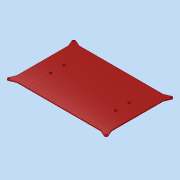
# Autodesk Inventor part: vna_mount
Saved by Autodesk Inventor 2022 (Build 260153000, 153)
## iProperties
Created: 2020-10-01
Part Number: vna_mount
Material: Generic
Document SubType Name: Modeling
Designer: nnico
Density: 1 g/cm^3
Appearance: Red
Author: nnico
Autodesk Inventor part; units mm, degrees
ref_plane "YZ Plane" through (0, 0, 0) normal (1, 0, 0) x (0, 1, 0)
ref_plane "XZ Plane" through (0, 0, 0) normal (0, 1, 0) x (-1, 0, 0)
ref_plane "XY Plane" through (0, 0, 0) normal (0, 0, 1) x (1, 0, 0)
sketch "Sketch1" plane through (0, 0, 0) normal (0, 1, 0) x (-1, 0, 0)
  line L0 (175, -115) -> (-175, -115)
  line L1 (-175, -115) -> (-175, 115)
  line L2 (-175, 115) -> (175, 115)
  line L3 (175, 115) -> (175, -115)
  line L4 (0, -115) -> (0, 115) construction
  line L5 (175, 0) -> (-175, 0) construction
  point P0 (0, 0)
  point P1 (0, 0)
  dimension "d0" = 350
  dimension "d1" = 230
  constraints: 12 end point, 5 midpoint, 2 parallel, 1 coincident, 1 horizontal, 1 perpendicular
  measures "d0" distance of L1.end L2.end
  measures "d1" distance of L0.end L1.end
extrude "Extrusion1" add sketch "Sketch1" along normal blind 3
sketch "Sketch2" plane through (0, 0, 0) normal (0, -1, 0) x (1, 0, 0)
  line L0 (175, -115) -> (-175, -115) construction
  line L1 (0, -115) -> (0, 115) construction
  line L2 (-175, 115) -> (175, 115) construction
  line L3 (130, -40) -> (110, -40)
  line L4 (110, -40) -> (110, 40)
  line L5 (110, 40) -> (130, 40)
  line L6 (130, 40) -> (130, -40)
  line L7 (130, 0) -> (110, 0) construction
  line L8 (0, 0) -> (175, 0) construction
  line L9 (175, 115) -> (175, -115) construction
  line L10 (-130, -40) -> (-110, -40)
  line L11 (-110, -40) -> (-110, 40)
  line L12 (-110, 40) -> (-130, 40)
  line L13 (-130, 40) -> (-130, -40)
  dimension "d4" = 20
  dimension "d5" = 80
  dimension "d6" = 220
  constraints: 22 end point, 5 midpoint, 4 symmetric about line, 2 parallel, 1 collinear, 1 horizontal, 1 perpendicular
  measures "d4" distance of L3.start L3.end
  measures "d5" distance of L5.end L3.start
  measures "d6" diameter of L3.end L1
extrude "Extrusion2" add sketch "Sketch2" along normal blind 10
sketch "Sketch3" plane through (0, -10, 0) normal (0, -1, 0) x (1, 0, 0)
  line L0 (175, 115) -> (-175, 115) construction
  line L1 (0, 115) -> (0, -115) construction
  line L2 (175, -115) -> (-175, -115) construction
  line L3 (0, 0) -> (-175, 0) construction
  line L4 (-175, 115) -> (-175, -115) construction
  line L5 (-110, 40) -> (-130, 40) construction
  line L6 (-120, 40) -> (-120, -40) construction
  line L7 (-130, -40) -> (-110, -40) construction
  circle A0 centre (-120, 25) radius 2.75
  circle A1 centre (-120, -25) radius 2.75
  circle A2 centre (120, 25) radius 2.75
  circle A3 centre (120, -25) radius 2.75
  dimension "d9" = 5.5
  dimension "d10" = 15
  constraints: 6 end point, 5 midpoint, 4 centre point, 3 symmetric about line, 1 point on line, 3 other
  measures "d9" diameter of A0
  measures "d10" distance from line of L5 A0.centre
extrude "Extrusion3" cut sketch "Sketch3" against normal up to next
sketch "Sketch4" plane through (0, 0, 0) normal (0, -1, 0) x (1, 0, 0)
  line L0 (110, 40) -> (110, -40) construction
  line L1 (110, 0) -> (-110, 0) construction
  line L2 (-110, -40) -> (-110, 40) construction
  line L3 (110, 15) -> (-110, 15)
  line L4 (-110, 15) -> (-110, 20)
  line L5 (-110, 20) -> (110, 20)
  line L6 (110, 20) -> (110, 15)
  line L7 (110, -15) -> (-110, -15)
  line L8 (-110, -15) -> (-110, -20)
  line L9 (-110, -20) -> (110, -20)
  line L10 (110, -20) -> (110, -15)
  point P0 (0, 0)
  dimension "d13" = 5
  dimension "d14" = 30
  constraints: 18 end point, 4 symmetric about line, 2 midpoint, 2 parallel, 2 point on line, 1 horizontal, 1 perpendicular
  measures "d13" distance of L3.end L4.end
  measures "d14" diameter of L3 L1
extrude "Extrusion4" add sketch "Sketch4" along normal blind 5
fillet "Fillet1" radius 10 6 edges at (120, 0, 40) (130, 0, 0) (120, 0, -40) (-120, 0, 40) (-130, 0, 0) (-120, 0, -40)
fillet "Fillet2" radius 5 4 edges at (0, 0, 20) (0, 0, -15) (0, 0, 15) (0, 0, -20)
sketch "Sketch5" plane through (0, 3, 0) normal (0, 1, 0) x (1, 0, 0)
  line L0 (-175, -115) -> (-175, 115) construction
  line L1 (-175, 0) -> (175, 0) construction
  line L2 (175, -115) -> (175, 115) construction
  line L3 (175, -115) -> (-175, -115) construction
  line L4 (0, -115) -> (0, 115) construction
  line L5 (-175, 115) -> (175, 115) construction
  circle A0 centre (-120, 25) radius 2.75 projected
  circle A1 centre (-120, 25) radius 4.5
  circle A2 centre (-120, -25) radius 4.5
  circle A3 centre (120, 25) radius 4.5
  circle A4 centre (120, -25) radius 4.5
  point P0 (0, 0)
  dimension "d19" = 9
  constraints: 4 centre point, 4 end point, 4 midpoint, 3 symmetric about line, 1 coincident, 3 other
  measures "d19" diameter of A1
extrude "Extrusion5" cut sketch "Sketch5" against normal blind 6
sketch "Sketch6" plane through (0, 3, 0) normal (0, 1, 0) x (1, 0, 0)
  line L0 (175, 115) -> (-175, 115) construction
  line L1 (0, 115) -> (0, -115) construction
  line L2 (175, -115) -> (-175, -115) construction
  line L3 (-175, 115) -> (-175, -115) construction
  line L4 (-175, 0) -> (175, 0) construction
  line L5 (175, -115) -> (175, 115) construction
  circle A0 centre (-179, 119) radius 6
  line L6 (-175, 115) -> (-179, 115) construction
  line L7 (-179, 115) -> (-179, 119) construction
  line L8 (-179, 119) -> (-175, 119) construction
  line L9 (-175, 119) -> (-175, 115) construction
  line L10 (-155, 115) -> (-175.4528, 123.8392)
  line L11 (-175, 95) -> (-183.0203, 114.5461)
  line L12 (-175, 95) -> (-175, 115)
  line L13 (-155, 115) -> (-175, 115)
  circle A1 centre (-179, -119) radius 6
  line L14 (-155, -115) -> (-175.4528, -123.8392)
  line L15 (-175, -95) -> (-183.0203, -114.5461)
  line L16 (-175, -95) -> (-175, -115)
  line L17 (-155, -115) -> (-175, -115)
  circle A2 centre (179, 119) radius 6
  line L18 (155, 115) -> (175.4528, 123.8392)
  line L19 (175, 95) -> (183.0203, 114.5461)
  line L20 (175, 95) -> (175, 115)
  line L21 (155, 115) -> (175, 115)
  line L22 (175, -95) -> (183.0203, -114.5461)
  circle A3 centre (179, -119) radius 6
  line L23 (155, -115) -> (175.4528, -123.8392)
  line L24 (155, -115) -> (175, -115)
  line L25 (175, -95) -> (175, -115)
  circle A4 centre (179, -119) radius 2.75
  circle A5 centre (179, 119) radius 2.75
  circle A6 centre (-179, -119) radius 2.75
  circle A7 centre (-179, 119) radius 2.75
  point P0 (0, 0)
  dimension "d22" = 12
  dimension "d23" = 4
  dimension "d24" = 4
  dimension "d25" = 20
  dimension "d26" = 20
  dimension "d30" = 5.5
  constraints: 44 end point, 17 symmetric about line, 8 centre point, 8 point on circle, 4 midpoint, 2 coincident, 2 collinear, 2 parallel, 2 point on line, 1 horizontal, 1 perpendicular, 6 other
  measures "d22" diameter of A0
  measures "d23" distance of L7.end L8.end
  measures "d24" distance of L6.end L7.end
  measures "d25" distance of L10.start L0.end
  measures "d26" distance of L11.start L0.end
  measures "d30" diameter of A4
extrude "Extrusion6" add sketch "Sketch6" against normal blind 3 contours A0 L13 L12 | A0 L10 L13 | A0 L12 L11 | A1 L16 L17 | L15 L16 A1 | A1 L17 L14 | A2 L20 L21 | A2 L21 L18 | L19 L20 A2 | L22 A3 L25 | A3 L24 L25 | A3 L23 L24 picked at (-175.087, 116.3056) picked at (-175.087, -116.3056) picked at (175.0917, 116.2969) picked at (175.0917, -116.2969)
body "Solid1"
